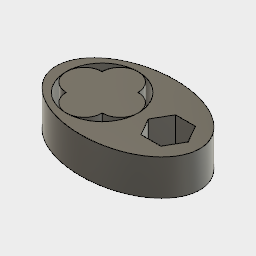
!-3 (Autodesk Fusion 360 archive; units mm, degrees)
design "模型3"
Autodesk Fusion 360 part; units mm, degrees
sketch "草图1" plane through (0, 0, 0) normal (0, 1, 0) x (1, 0, 0)
  ellipse E0 centre (-3.7384, -6.0454) end of major axis (46.2616, -6.0454) minor radius 33
  circle A0 centre (-21.7384, -6.0454) radius 25
  line L0 (17.3334, 5.9546) -> (31.1898, 5.9546)
  line L1 (14.987, -18.0454) -> (31.1898, -18.0454)
  line L2 (31.1898, 5.9546) -> (38.118, -6.0454)
  line L3 (31.1898, -18.0454) -> (38.118, -6.0454)
  line L4 (17.3334, 5.9546) -> (10.4052, -6.0454)
  line L5 (10.4052, -6.0454) -> (17.3334, -18.0454)
  line L6 (-53.7384, -6.0454) -> (10.4052, -6.0454) construction
  line L7 (38.118, -6.0454) -> (46.2616, -6.0454) construction
  line L8 (-3.7384, -39.0454) -> (-3.7384, -23.3947) construction
  line L9 (-3.7384, 11.304) -> (-3.7384, 26.9546) construction
  arc A1 (-34.2384, 6.4546) -> (-34.2384, -18.5454) centre (-34.2384, -6.0454) ccw
  arc A2 (-9.2384, 6.4546) -> (-34.2384, 6.4546) centre (-21.7384, 6.4546) ccw
  arc A3 (-34.2384, -18.5454) -> (-9.2384, -18.5454) centre (-21.7384, -18.5454) ccw
  arc A4 (-9.2384, -18.5454) -> (-9.2384, 6.4546) centre (-9.2384, -6.0454) ccw
  dimension "d1" = 100
  dimension "d2" = 66
  dimension "d4" = 50
  measures "d1" distance of E0
  measures "d4" diameter of A0
extrude "拉伸1" add sketch "草图1" along normal blind 10 contours E0 | A1 A2 A3 A4
extrude "拉伸2" add 2 faces at (8.5366, 10, -13.0979) (-25.9051, 10, 1.8787) along direction (0, 1, 0) blind 15
